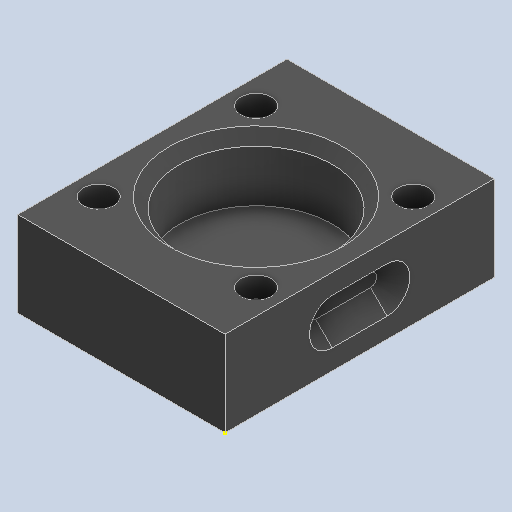
# Autodesk Inventor part: Pieza1
Saved by Autodesk Inventor 2026 (Build 300175050, 175E)
## iProperties
Created: 2025-09-26
Part Number: Pieza1
Material: Plastico PETG
Document SubType Name: Modeling
Designer: bello
Density: 1.27 g/cm^3
Appearance: Genérico
Author: bello
Autodesk Inventor part; units mm, degrees
ref_plane "YZ Plane" through (0, 0, 0) normal (1, 0, 0) x (0, 1, 0)
ref_plane "XZ Plane" through (0, 0, 0) normal (0, 1, 0) x (-1, 0, 0)
sketch "Boceto1" plane through (0, 0, 0) normal (0, 1, 0) x (-1, 0, 0)
  line L0 (0, 0) -> (-50.2, 0)
  line L1 (-50.2, 0) -> (-50.2, -65.2)
  line L2 (-50.2, -65.2) -> (0, -65.2)
  line L3 (0, -65.2) -> (0, 0)
  dimension "d0" = 50.2
  dimension "d1" = 65.2
  constraints: 8 end point, 2 parallel, 1 horizontal, 1 perpendicular
  measures "d0" distance of L2.end L1.end
  measures "d1" distance of L0.end L1.end
extrude "Extrusión1" add sketch "Boceto1" along normal blind 20.7
sketch "Boceto2" plane through (0, 20.7, 0) normal (0, 1, 0) x (1, 0, 0)
  line L0 (-14.4985, 32.6) -> (58.2485, 32.6)
  circle A0 centre (25.1, 32.6) radius 18.5
  line L1 (0, 65.2) -> (0, 0) projected
  dimension "d7" = 37
  dimension "d57" = 0
  dimension "d58" = 25.1
  constraints: 2 end point, 2 horizontal, 1 centre point
  measures "d7" diameter of A0
  measures "d57" distance from line of A0.centre L0
  measures "d58" distance from line of L1 A0.centre
extrude "Extrusión2" cut sketch "Boceto2" against normal blind 15
sketch "Boceto3" plane through (50.2, 0, 0) normal (1, 0, 0) x (0, 0, -1)
  line L0 (32.6, 28.8672) -> (32.6, -9.3744)
  line L1 (-5.2256, 10.35) -> (70.0589, 10.35)
  line L2 (25.95, 10.35) -> (39.25, 10.35) construction
  line L3 (25.95, 8.85) -> (39.25, 8.85)
  line L4 (39.25, 11.85) -> (25.95, 11.85)
  arc A0 (25.95, 11.85) -> (25.95, 8.85) centre (25.95, 10.35) ccw
  arc A1 (39.25, 8.85) -> (39.25, 11.85) centre (39.25, 10.35) ccw
  point P0 (0, 0)
  point P1 (32.6, 10.35)
  point P2 (40.75, 10.35)
  point P3 (24.45, 10.35)
  dimension "d11" = 16.3
  dimension "d12" = 3
  dimension "d13" = 0
  constraints: 12 end point, 6 point on circle, 4 tangent, 2 centre point, 2 horizontal, 2 point on line, 2 vertical, 1 midpoint, 1 parallel
  measures "d11" distance of point (40.75, 10.35) point (24.45, 10.35)
  measures "d12" distance between parallel lines of L3 L4
  measures "d13" distance from line of point (32.6, 10.35) L0
extrude "Extrusión3" cut sketch "Boceto3" against normal blind 4
chamfer "Chaflán1" distance 4 angle 45 4 edges at (50.2, 8.85, -32.6) (50.2, 10.35, -24.45) (50.2, 11.85, -32.6) (50.2, 10.35, -40.75)
sketch "Boceto4" plane through (50.2, 0, 0) normal (1, 0, 0) x (0, 0, -1)
  point P0 (0, 0)
ref_plane "Plano de trabajo1" through (25.1, 0, 0) normal (1, 0, 0) x (0, 0, -1)
mirror "Simetría1" about plane through (25.1, 0, 0) normal (1, 0, 0) of "Extrusión3"
chamfer "Chaflán2" distance 4 angle 45 4 edges at (0, 11.85, -32.6) (0, 10.35, -24.45) (0, 8.85, -32.6) (0, 10.35, -40.75)
chamfer "Chaflán3" distance 2.5 angle 45 1 edges at (6.6, 20.7, -32.6)
sketch "Boceto5" plane through (0, 0, 0) normal (0, -1, 0) x (1, 0, 0)
  line L0 (25.1, 22.2035) -> (25.1, -86.3829)
  line L1 (-10.0483, -32.6) -> (59.9656, -32.6)
  circle A0 centre (6.05, -7.2) radius 3.2
  circle A1 centre (44.15, -7.2) radius 3.2
  circle A2 centre (6.05, -58) radius 3.2
  circle A3 centre (31.45, -45.3) radius 3.2
  point P0 (0, 0)
  dimension "d35" = 38.1
  dimension "d36" = 38.1
  dimension "d37" = 0
  dimension "d38" = 50.8
  dimension "d39" = 50.8
  dimension "d40" = 12.7
  dimension "d41" = 12.7
  dimension "d42" = 6.4
  constraints: 4 centre point, 4 end point, 3 equal radius, 2 horizontal, 2 vertical
  measures "d35" distance of A0.centre A1.centre
  measures "d36" diameter of A0.centre L0
  measures "d37" horizontal distance of A2.centre A0.centre
  measures "d38" distance of A0.centre A2.centre
  measures "d39" diameter of A0.centre L1
  measures "d40" vertical distance of A2.centre A3.centre
  measures "d41" horizontal distance of A3.centre A1.centre
  measures "d42" diameter of A0
extrude "Extrusión4" add sketch "Boceto5" along normal blind 4.2
fillet "Empalme1" radius 3.2 4 edges at (2.85, -4.2, -58) (28.25, -4.2, -45.3) (40.95, -4.2, -7.2) (2.85, -4.2, -7.2)
sketch "Boceto6" plane through (0, 20.7, 0) normal (0, 1, 0) x (1, 0, 0)
  line L0 (-6.6573, 32.6) -> (60.5927, 32.6)
  line L1 (25.1, -18.2708) -> (25.1, 82.1469)
  circle A0 centre (6.05, 13.55) radius 3.7
  circle A1 centre (6.05, 51.65) radius 3.7
  circle A2 centre (44.15, 13.55) radius 3.7
  circle A3 centre (44.15, 51.65) radius 3.7
  point P0 (0, 0)
  dimension "d51" = 38.1
  dimension "d52" = 38.1
  dimension "d53" = 38.1
  dimension "d54" = 38.1
  dimension "d55" = 38.1
  dimension "d56" = 7.4
  constraints: 4 centre point, 4 end point, 3 equal radius, 2 horizontal, 2 vertical
  measures "d51" distance of A0.centre A1.centre
  measures "d52" diameter of A0.centre L0
  measures "d53" distance of A0.centre A2.centre
  measures "d54" diameter of A0.centre L1
  measures "d55" diameter of A3.centre L1
  measures "d56" diameter of A2
extrude "Extrusión5" cut sketch "Boceto6" against normal blind 5
